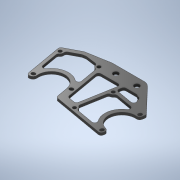
# Autodesk Inventor part: Knee_side_frame
Saved by Autodesk Inventor 2022 (Build 260153000, 153)
## iProperties
Part Number: Knee_side_frame
Material: アルミニウム 2014-T4
Document SubType Name: Modeling
Designer: Masato Kubotera
Density: 2.8 g/cm^3
Appearance: Smooth - Black
Description: A2017 T2
Mass: 7.47673 g
Surface Area: 40.0753 cm^2
Volume: 2.67026 cm^3
Author: Masato Kubotera
Revision Number: Rev.2 Specifications for RoboCup 2023: Anodized aluminum staining process added.
Autodesk Inventor part; units mm, degrees
ref_plane "YZ Plane" through (0, 0, 0) normal (1, 0, 0) x (0, 1, 0)
ref_plane "XZ Plane" through (0, 0, 0) normal (0, 1, 0) x (-1, 0, 0)
ref_plane "XY Plane" through (0, 0, 0) normal (0, 0, 1) x (1, 0, 0)
sketch "スケッチ1" plane through (0, 0, 0) normal (0, 0, 1) x (1, 0, 0)
  line L0 (-46.5961, 42.1731) -> (-4.2493, 49.64) construction
  line L1 (-4.2493, 49.64) -> (1.3074, 18.1262) construction
  line L2 (1.3074, 18.1262) -> (-41.0393, 10.6593) construction
  line L3 (-41.0393, 10.6593) -> (-46.5961, 42.1731) construction
  line L4 (-46.5961, 42.1731) -> (1.3074, 18.1262) construction
  line L5 (-4.2493, 49.64) -> (-41.0393, 10.6593) construction
  line L6 (-43.8177, 26.4162) -> (-1.471, 33.8831) construction
  line L7 (-6.7696, 46.6571) -> (-33.3594, 41.9686) construction
  line L8 (-33.3594, 41.9686) -> (-28.6709, 15.3787) construction
  line L9 (-28.6709, 15.3787) -> (-2.0811, 20.0672) construction
  line L10 (-2.0811, 20.0672) -> (-6.7696, 46.6571) construction
  line L11 (-6.7696, 46.6571) -> (-28.6709, 15.3787) construction
  line L12 (-33.3594, 41.9686) -> (-2.0811, 20.0672) construction
  circle A0 centre (-32, 28.5) radius 10.5 construction
  line L13 (-20.0645, 44.3128) -> (-15.376, 17.723) construction
  circle A1 centre (-6.7696, 46.6571) radius 1.35
  circle A2 centre (-2.0811, 20.0672) radius 1.35
  arc A3 (-36.1041, 41.4846) -> (-33.0796, 39.1957) centre (-33.3594, 41.9686) ccw
  line L14 (-36.1041, 41.4846) -> (-36.5382, 43.9466)
  circle A4 centre (0, 8.5) radius 2.05
  circle A5 centre (0, 8.5) radius 6 construction
  circle A6 centre (0, 8.5) radius 4.6 construction
  line L15 (-36.5382, 43.9466) -> (-4.2493, 49.64)
  circle A7 centre (-32, -28.5) radius 10.5 construction
  line L16 (-31.7738, 42.2481) -> (-9.2317, 46.2229)
  arc A8 (-27.0853, 15.6583) -> (-31.7738, 42.2481) centre (-32, 28.5) ccw
  line L17 (-27.0853, 15.6583) -> (-4.5432, 19.6331)
  arc A9 (-9.2317, 46.2229) -> (-5.0921, 44.8035) centre (-6.7696, 46.6571) ccw
  arc A10 (-1.1387, 22.3828) -> (-4.5432, 19.6331) centre (-2.0811, 20.0672) ccw
  arc A11 (-32.03, 42.203) -> (-34.6889, 41.7341) centre (-33.3594, 41.9686) ccw
  arc A12 (-34.6021, 41.2417) -> (-31.9431, 41.7106) centre (-33.2726, 41.4761) ccw
  line L18 (-34.6889, 41.7341) -> (-34.6021, 41.2417)
  line L19 (-31.9431, 41.7106) -> (-32.03, 42.203)
  arc A13 (-30.0004, 15.1443) -> (-27.3415, 15.6132) centre (-28.6709, 15.3787) ccw
  arc A14 (-27.4283, 16.1056) -> (-30.0873, 15.6367) centre (-28.7578, 15.8711) ccw
  line L20 (-30.0004, 15.1443) -> (-30.0873, 15.6367)
  line L21 (-27.4283, 16.1056) -> (-27.3415, 15.6132)
  line L22 (-49.8407, -37.5393) -> (-42.3738, 4.8074) construction
  line L23 (-42.3738, 4.8074) -> (-10.86, -0.7493) construction
  line L24 (-10.86, -0.7493) -> (-18.3269, -43.0961) construction
  line L25 (-18.3269, -43.0961) -> (-49.8407, -37.5393) construction
  line L26 (-49.8407, -37.5393) -> (-10.86, -0.7493) construction
  line L27 (-42.3738, 4.8074) -> (-18.3269, -43.0961) construction
  line L28 (-34.0838, -40.3177) -> (-26.6169, 2.029) construction
  line L29 (-18.5314, -29.8594) -> (-13.8429, -3.2696) construction
  line L30 (-13.8429, -3.2696) -> (-40.4328, 1.4189) construction
  line L31 (-40.4328, 1.4189) -> (-45.1213, -25.1709) construction
  line L32 (-45.1213, -25.1709) -> (-18.5314, -29.8594) construction
  line L33 (-18.5314, -29.8594) -> (-40.4328, 1.4189) construction
  line L34 (-13.8429, -3.2696) -> (-45.1213, -25.1709) construction
  circle A15 centre (-40.4328, 1.4189) radius 1.35
  arc A16 (-44.8868, -23.8415) -> (-45.3557, -26.5004) centre (-45.1213, -25.1709) ccw
  line L35 (-44.8868, -23.8415) -> (-44.3944, -23.9283)
  line L36 (-44.8633, -26.5873) -> (-45.3557, -26.5004)
  arc A17 (-44.8633, -26.5873) -> (-44.3944, -23.9283) centre (-44.6289, -25.2578) ccw
  line L37 (-32, -28.5) -> (-32, 28.5) construction
  line L38 (-13.8429, -3.2696) -> (-18.5314, -29.8594) construction
  circle A18 centre (-13.8429, -3.2696) radius 1.35
  arc A19 (-18.7659, -31.1889) -> (-18.297, -28.53) centre (-18.5314, -29.8594) ccw
  line L39 (-18.297, -28.53) -> (-18.7894, -28.4431)
  line L40 (-19.2583, -31.1021) -> (-18.7659, -31.1889)
  arc A20 (-18.7894, -28.4431) -> (-19.2583, -31.1021) centre (-19.0239, -29.7726) ccw
  circle A21 centre (0, -8.5) radius 2.05
  circle A22 centre (0, -8.5) radius 6 construction
  line L41 (0, 8.5) -> (0, -8.5) construction
  arc A23 (-30.1333, 17.9133) -> (-33.0796, 39.1957) centre (-32, 28.5) ccw
  arc A24 (-21.3013, -29.5493) -> (-42.4123, -25.8268) centre (-32, -28.5) ccw
  arc A25 (-20.4814, -20.991) -> (-40.2557, -17.5043) centre (-32, -28.5) ccw
  line L42 (-47.9807, -26.9905) -> (-45.0262, -27.5114)
  arc A26 (-45.0262, -27.5114) -> (-42.4123, -25.8268) centre (-44.6289, -25.2578) ccw
  arc A27 (-21.3013, -29.5493) -> (-19.4212, -32.0263) centre (-19.0239, -29.7726) ccw
  line L43 (-16.4668, -32.5472) -> (4.1466, -12.8365)
  line L44 (6, -8.5) -> (6, 17.4276)
  arc A28 (4.1466, -12.8365) -> (6, -8.5) centre (0, -8.5) ccw
  arc A29 (-39.7274, -0.9796) -> (-38.2562, 0.1889) centre (-40.4328, 1.4189) ccw
  line L45 (-43.4262, -15.5576) -> (-41.1328, -2.551)
  line L46 (-36.1677, 1.1745) -> (-17.9343, -2.0405)
  arc A30 (-16.3089, -3.681) -> (-15.3261, -5.2822) centre (-13.8429, -3.2696) ccw
  line L47 (-16.8364, -20.2461) -> (-14.5429, -7.2395)
  line L48 (-11.6414, -5.181) -> (-13.7929, -17.3828)
  circle A31 centre (-13.8429, -3.2696) radius 2.4 construction
  arc A32 (-41.98, 15.994) -> (-29.2216, 12.7431) centre (-32, 28.5) ccw construction
  line L49 (-40.7981, 4.5296) -> (-39.3221, 12.9004) construction
  line L50 (-39.3221, 12.9004) -> (-10.9597, 7.8994) construction
  line L51 (-12.4357, -0.4715) -> (-10.9597, 7.8994) construction
  line L52 (-19.4212, -32.0263) -> (-16.4668, -32.5472)
  line L53 (-47.9807, -26.9905) -> (-40.3815, 16.1063)
  line L54 (-40.3815, 16.1063) -> (-30.1333, 17.9133)
  arc A33 (-11.3809, -3.7038) -> (-11.3438, -3.2026) centre (-13.8429, -3.2696) ccw
  line L55 (-9.3245, -3.5586) -> (-7.6527, -3.8534)
  line L56 (-35.8308, 10.2414) -> (-36.6101, 5.822)
  line L57 (-34.9878, 3.505) -> (-8.3473, -1.1924)
  line L58 (-6, 0.7772) -> (-6, 14.4542)
  line L59 (-34.2085, 11.8638) -> (-8.3473, 16.4238)
  arc A34 (-43.4262, -15.5576) -> (-40.2557, -17.5043) centre (-41.4566, -15.9049) ccw
  arc A35 (-20.4814, -20.991) -> (-16.8364, -20.2461) centre (-18.806, -19.8988) ccw
  line L60 (-6, -5.823) -> (-6, -14.0743)
  line L61 (-4.2493, 49.64) -> (2.6187, 36.6039)
  line L62 (-1.2105, 32.4059) -> (0.2667, 32.6664) construction
  line L63 (0.2667, 32.6664) -> (-0.2542, 35.6208)
  line L64 (-0.2542, 35.6208) -> (-1.7314, 35.3603) construction
  line L65 (-0.2542, 35.6208) -> (-5.0921, 44.8035)
  line L66 (0.2667, 32.6664) -> (-1.1387, 22.3828)
  line L67 (2.6187, 36.6039) -> (6, 17.4276)
  line L68 (-8.1997, -18.416) -> (-7.477, -17.7249)
  line L69 (-10.4411, -19.1756) -> (-10.4411, -19.1756)
  line L70 (-6.6178, -15.5198) -> (-6.6178, -15.5198)
  arc A36 (-34.2085, 11.8638) -> (-35.8308, 10.2414) centre (-33.8612, 9.8941) ccw
  arc A37 (-36.6101, 5.822) -> (-34.9878, 3.505) centre (-34.6405, 5.4747) ccw
  arc A38 (-8.3473, -1.1924) -> (-6, 0.7772) centre (-8, 0.7772) ccw
  arc A39 (-6, 14.4542) -> (-8.3473, 16.4238) centre (-8, 14.4542) ccw
  arc A40 (-39.7274, -0.9796) -> (-41.1328, -2.551) centre (-39.1631, -2.8983) ccw
  arc A41 (-36.1677, 1.1745) -> (-38.2562, 0.1889) centre (-36.515, -0.7951) ccw
  arc A42 (-16.3089, -3.681) -> (-17.9343, -2.0405) centre (-18.2816, -4.0101) ccw
  arc A43 (-14.5429, -7.2395) -> (-15.3261, -5.2822) centre (-16.5126, -6.8922) ccw
  arc A44 (-9.3245, -3.5586) -> (-11.6414, -5.181) centre (-9.6718, -5.5283) ccw
  arc A45 (-13.7929, -17.3828) -> (-10.4411, -19.1756) centre (-11.8233, -17.7301) ccw
  arc A46 (-6.6178, -15.5198) -> (-6, -14.0743) centre (-8, -14.0743) ccw
  arc A47 (-6, -5.823) -> (-7.6527, -3.8534) centre (-8, -5.823) ccw
  arc A48 (-9.0001, -18.6873) -> (-8.1997, -18.416) centre (-8.8908, -17.6932) ccw
  arc A49 (-7.477, -17.7249) -> (-7.1702, -16.9375) centre (-8.1681, -17.0021) ccw
  arc A50 (-9.0001, -18.6873) -> (-10.4411, -19.1756) centre (-9.1968, -20.4769) ccw
  arc A51 (-6.6178, -15.5198) -> (-7.1702, -16.9375) centre (-5.3735, -16.821) ccw
  point P0 (-22.6443, 30.1497)
  point P1 (-17.7203, 31.0179)
  point P2 (-30.3503, -19.1443)
  point P3 (-29.4821, -14.2203)
  point P4 (-29.4821, -14.2203)
  point P5 (-44.8417, -23.5853)
  point P6 (6, 8.5)
  point P7 (-40.8669, -1.0432)
  point P8 (-14.8529, -23.3942)
  point P9 (-37.9337, 1.4859)
  point P10 (-16.1684, -2.3519)
  point P11 (-14.2771, -5.7317)
  point P12 (-18.2519, -28.2738)
  point P13 (-13.0711, -52.3219)
  point P14 (-12.9341, -52.334)
  point P15 (13.7499, -57.0391)
  point P16 (13.8829, -57.0746)
  point P17 (-6, -4.1448)
  point P18 (-6, -14.929)
  point P19 (-35.5876, 11.6206)
  point P20 (-36.9574, 3.8523)
  point P21 (-6, -1.6063)
  point P22 (-6, 16.8377)
  point P23 (0, 0)
  point P24 (0, 0)
  point P25 (-8.9225, -19.1071)
  point P26 (-6.7542, -17.0338)
  point P27 (-7.4453, -16.311)
  point P28 (-9.6136, -18.3844)
  point P29 (-9.6136, -18.3844)
  point P30 (-7.4453, -16.311)
  point P31 (-9.1917, -17.981)
  point P32 (-7.0235, -15.9077)
  point P33 (-10.4411, -19.1756)
  dimension "d34" = 12
  dimension "d21" = 43
  dimension "d22" = 32
  dimension "d23" = 27
  dimension "d24" = 27
  dimension "d27" = 21
  dimension "d28" = 9.5
  dimension "d31" = 4.1
  dimension "d39" = 8.5
  dimension "d40" = 9.2
  dimension "d41" = 32
  dimension "d46" = 20
  dimension "d56" = 2.5
  dimension "d57" = 2.5
  dimension "d63" = 2.5
  dimension "d67" = 2.7
  dimension "d68" = 1.35
  dimension "d70" = 0.5
  dimension "d72" = 43
  dimension "d73" = 32
  dimension "d77" = 9.5
  dimension "d78" = 20
  dimension "d80" = 27
  dimension "d81" = 27
  dimension "d82" = 8.5
  dimension "d83" = 2.7
  dimension "d86" = 0.5
  dimension "d87" = 1.35
  dimension "d88" = 57
  dimension "d89" = 80
  dimension "d90" = 21
  dimension "d91" = 100
  dimension "d92" = 4.1
  dimension "d93" = 12
  dimension "d94" = 17
  dimension "d95" = 3
  dimension "d96" = 0.25
  dimension "d97" = 0.25
  dimension "d98" = 3
  dimension "d99" = 0
  dimension "d101" = 2.5
  dimension "d107" = 2.5
  dimension "d109" = 2.5
  dimension "d111" = 4.8
  dimension "d112" = 8.5
  dimension "d113" = 28.8
  dimension "d114" = 2.5
  dimension "d115" = 2.5
  dimension "d116" = 2
  dimension "d117" = 2
  dimension "d118" = 2.5
  dimension "d119" = 5.5
  dimension "d120" = 2.5
  dimension "d121" = 1.5
  dimension "d122" = 3
  dimension "d123" = 3
  dimension "d125" = 3
  dimension "d126" = 1
  dimension "d127" = 3
  dimension "d130" = 2
  dimension "d131" = 2
  dimension "d132" = 2
  dimension "d133" = 1
  dimension "d136" = 4.5
  constraints: 142 end point, 90 point on circle, 52 tangent, 51 centre point, 43 point on line, 27 parallel, 24 coincident, 22 symmetric about line, 16 midpoint, 13 perpendicular, 11 equal radius, 5 vertical, 3 collinear, 1 horizontal alignment, 26 other
  measures "d21" distance of L1.end L2.end
  measures "d22" distance of L0.end L1.end
  measures "d23" distance of L9.end L8.end
  measures "d24" distance of L8.end L7.end
  measures "d27" diameter of A0
  measures "d28" distance of point (-22.644, 30.15) A0.centre
  measures "d31" diameter of A4
  measures "d39" distance from line of L8 point (-22.644, 30.15)
  measures "d40" diameter of A6
  measures "d41" horizontal distance of A4.centre A0.centre
  measures "d46" vertical distance of L41.start A0.centre
  measures "d56" radius of A9
  measures "d57" distance from line of L16.end L15
  measures "d63" radius of A10
  measures "d67" diameter of A1
  measures "d68" radius of A11
  measures "d70" distance of L19.start L19.end
  measures "d72" distance of L23.end L24.end
  measures "d73" distance of L22.end L23.end
  measures "d77" distance of L37.start point (-30.35, -19.144)
  measures "d78" angle of L23 L2
  measures "d80" distance of L29.start L29.end
  measures "d81" distance of L29.end L30.end
  measures "d82" distance from line of L32 point (-30.35, -19.144)
  measures "d83" diameter of A15
  measures "d86" distance of L31.end A17.centre
  measures "d87" radius of A16
  measures "d88" distance of L37.start A0.centre
  measures "d89" angle of L37 L2
  measures "d90" diameter of A7
  measures "d91" angle of L23 L37
  measures "d92" diameter of A21
  measures "d93" diameter of A22
  measures "d94" distance of L41.start L41.end
  measures "d95" radial gap between concentric circles of A23 A8
  measures "d96" radial gap between concentric circles of A0 A23
  measures "d97" radial gap between concentric circles of A7 A24
  measures "d98" radial gap between concentric circles of A24 A25
  measures "d99" distance between parallel lines of L9 L17
  measures "d101" radius of A29
  measures "d107" distance between parallel lines of L46 L23
  measures "d109" distance between parallel lines of L47 L48
  measures "d111" diameter of A31
  measures "d112" distance of L49.start L49.end
  measures "d113" distance of L49.end L50.end
  measures "d114" distance between parallel lines of L53 L45
  measures "d115" radius of A33
  measures "d116" radius of A34
  measures "d117" radius of A35
  measures "d118" distance between parallel lines of L46 L57
  measures "d119" distance between parallel lines of L53 L56
  measures "d120" distance between parallel lines of L59 L17
  measures "d121" distance of L63.end L64.end
  measures "d122" distance of L62.end L63.end
  measures "d123" distance between parallel lines of L65 L61
  measures "d125" distance between parallel lines of L67 L63
  measures "d126" distance of point (-6.754, -17.034) point (-7.445, -16.311)
  measures "d127" distance of point (-8.922, -19.107) point (-6.754, -17.034)
  measures "d130" radius of A36
  measures "d131" radius of A40
  measures "d132" radius of A44
  measures "d133" radius of A48
  measures "d136" distance between parallel lines of L43 L68
extrude "押し出し1" add sketch "スケッチ1" along normal blind 2
fillet "フィレット1" radius 2 8 edges at (-36.5382, 43.9466, 1) (-4.2493, 49.64, 1) (-16.4668, -32.5472, 1) (-47.9807, -26.9905, 1) (-30.1333, 17.9133, 1) (-40.3815, 16.1063, 1) (2.6187, 36.6039, 1) (6, 17.4276, 1)
fillet "フィレット2" radius 2 8 edges at (-31.7738, 42.2481, 1) (-27.0853, 15.6583, 1) (-4.5432, 19.6331, 1) (-9.2317, 46.2229, 1) (0.2667, 32.6664, 1) (-0.2542, 35.6208, 1) (-1.1387, 22.3828, 1) (-5.0921, 44.8035, 1)
